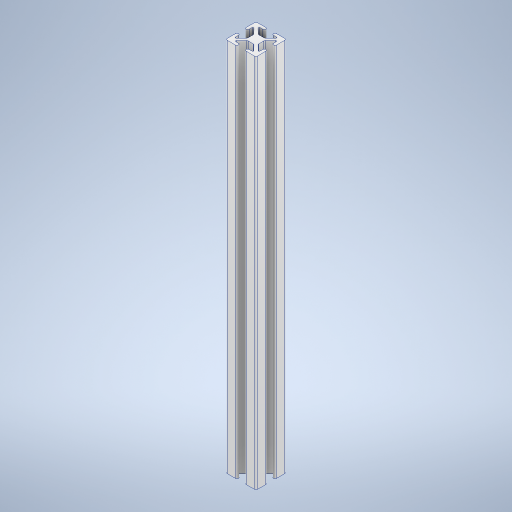
# Autodesk Inventor part: T_slot_1in_12.35in
Saved by Autodesk Inventor 2024 (Build 280153000, 153)
## iProperties
Created: 2024-09-19
Part Number: T_slot_1in_12.35in
Material: Aluminum 6061
Document SubType Name: Modeling
Designer: Owner
Density: 2.7 g/cm^3
Appearance: Aluminum - Flat
Author: Owner
Autodesk Inventor part; units mm, degrees
ref_plane "YZ Plane" through (0, 0, 0) normal (1, 0, 0) x (0, 1, 0)
ref_plane "XZ Plane" through (0, 0, 0) normal (0, 1, 0) x (-1, 0, 0)
ref_plane "XY Plane" through (0, 0, 0) normal (0, 0, 1) x (1, 0, 0)
sketch "Sketch1" plane through (0, 0, 0) normal (0, 1, 0) x (-1, 0, 0)
  line L0 (12.7, 12.7) -> (-12.7, 12.7)
  line L1 (-12.7, 12.7) -> (-12.7, -12.7)
  line L2 (-12.7, -12.7) -> (12.7, -12.7)
  line L3 (12.7, -12.7) -> (12.7, 12.7)
  line L4 (12.7, 12.7) -> (-12.7, -12.7) construction
  line L5 (-12.7, 12.7) -> (12.7, -12.7) construction
  line L6 (10.16, 10.16) -> (-10.16, 10.16)
  line L7 (-10.16, 10.16) -> (-10.16, -10.16)
  line L8 (-10.16, -10.16) -> (10.16, -10.16)
  line L9 (10.16, -10.16) -> (10.16, 10.16)
  line L10 (10.16, 10.16) -> (-10.16, -10.16) construction
  line L11 (-10.16, 10.16) -> (10.16, -10.16) construction
  line L12 (-4.445, 4.445) -> (4.445, 4.445)
  line L13 (4.445, 4.445) -> (4.445, -4.445)
  line L14 (4.445, -4.445) -> (-4.445, -4.445)
  line L15 (-4.445, -4.445) -> (-4.445, 4.445)
  line L16 (-4.445, 4.445) -> (4.445, -4.445) construction
  line L17 (4.445, 4.445) -> (-4.445, -4.445) construction
  line L18 (0, 12.7) -> (-3.175, 12.7)
  line L19 (-3.175, 12.7) -> (3.175, 12.7)
  line L20 (3.175, 12.7) -> (3.175, -12.7)
  line L21 (3.175, -12.7) -> (-3.175, -12.7)
  line L22 (-3.175, -12.7) -> (-3.175, 12.7)
  line L23 (12.7, 0) -> (12.7, 3.175)
  line L24 (12.7, 3.175) -> (-12.7, 3.175)
  line L25 (-12.7, 3.175) -> (-12.7, -3.175)
  line L26 (-12.7, -3.175) -> (12.7, -3.175)
  line L27 (12.7, -3.175) -> (12.7, 3.175)
  line L28 (-13.598, -11.802) -> (11.802, 13.598)
  line L29 (11.802, 13.598) -> (13.598, 11.802)
  line L30 (13.598, 11.802) -> (-11.802, -13.598)
  line L31 (-11.802, -13.598) -> (-13.598, -11.802)
  line L32 (-13.598, -11.802) -> (13.598, 11.802) construction
  line L33 (11.802, 13.598) -> (-11.802, -13.598) construction
  line L34 (-13.598, 11.802) -> (11.802, -13.598)
  line L35 (11.802, -13.598) -> (13.598, -11.802)
  line L36 (13.598, -11.802) -> (-11.802, 13.598)
  line L37 (-11.802, 13.598) -> (-13.598, 11.802)
  line L38 (-13.598, 11.802) -> (13.598, -11.802) construction
  line L39 (11.802, -13.598) -> (-11.802, 13.598) construction
  point P0 (0, 0)
  point P1 (8.3639, 10.16)
  point P2 (2.6489, 4.445)
  point P3 (-2.6489, 4.445)
  point P4 (-8.3639, 10.16)
  point P5 (-10.16, 3.175)
  point P6 (-10.16, 8.3639)
  point P7 (-4.445, 2.6489)
  point P8 (-4.445, -2.6489)
  point P9 (-10.16, -8.3639)
  point P10 (-10.16, -3.175)
  point P11 (-3.175, -10.16)
  point P12 (-8.3639, -10.16)
  point P13 (-2.6489, -4.445)
  point P14 (2.6489, -4.445)
  point P15 (8.3639, -10.16)
  point P16 (3.175, -10.16)
  point P17 (10.16, -3.175)
  point P18 (10.16, -8.3639)
  point P19 (4.445, -2.6489)
  point P20 (4.445, 2.6489)
  point P21 (10.16, 8.3639)
  point P22 (10.16, 3.175)
  point P23 (-3.175, 10.16)
  point P24 (3.175, 10.16)
  dimension "d0" = 25.4
  dimension "d1" = 25.4
  dimension "d2" = 20.32
  dimension "d3" = 20.32
  dimension "d4" = 8.89
  dimension "d5" = 8.89
  dimension "d6" = 3.175
  dimension "d7" = 6.35
  dimension "d8" = 3.175
  dimension "d9" = 6.35
  dimension "d10" = 2.54
  dimension "d11" = 2.54
  constraints: 80 end point, 16 parallel, 12 midpoint, 7 perpendicular, 5 horizontal, 4 point on line
  measures "d0" distance of L2.end L1.end
  measures "d1" distance of L1.end L0.end
  measures "d2" distance of L8.end L7.end
  measures "d3" distance of L7.end L6.end
  measures "d4" distance of L13.end L14.end
  measures "d5" distance of L12.end L13.end
  measures "d6" distance of L18.start L18.end
  measures "d7" distance of L20.end L21.end
  measures "d8" distance of L23.start L23.end
  measures "d9" distance of L25.end L24.end
  measures "d10" distance of L28.end L29.end
  measures "d11" distance of L35.end L34.end
extrude "Extrusion1" add sketch "Sketch1" along normal blind 313.69 contours L0 L28 L6 L20 | L0 L3 L30 L9 L6 L28 | L22 L6 L36 L0 | L6 L9 L30 L24 L13 L12 L20 L28 | L20 L12 L28 | L36 L6 L7 L34 L1 L0 | L3 L24 L9 L30 | L36 L22 L12 L15 L24 L34 L7 L6 | L36 L12 L22 | L20 L24 L28 L12 | L12 L13 L24 L20 | L28 L24 L36 L12 | L22 L24 L15 L12 | L12 L36 L24 L22 | L24 L13 L30 L20 | L20 L30 L36 L28 L24 | L28 L36 L24 | L34 L7 L24 L1 | L30 L13 L24 | L24 L36 L28 L34 L22 | L22 L34 L15 L24 | L30 L13 L36 L20 | L20 L36 L30 | L36 L30 L34 L28 | L3 L36 L9 L26 | L24 L15 L34 | L34 L28 L22 | L22 L28 L15 L34 | L36 L13 L26 L20 | L20 L26 L34 L30 L36 | L34 L30 L26 L22 L28 | L26 L7 L28 L1 | L3 L2 L34 L8 L9 L36 | L9 L8 L34 L20 L14 L13 L26 L36 | L26 L13 L36 | L22 L26 L15 L28 | L26 L13 L14 L20 | L20 L14 L34 L26 | L34 L26 L30 | L28 L7 L8 L30 L2 L1 | L28 L26 L15 L14 L22 L30 L8 L7 | L28 L15 L26 | L26 L30 L14 L22 | L22 L14 L15 L26 | L20 L34 L14 | L34 L14 L30 L26 | L2 L20 L8 L34 | L14 L30 L22 | L30 L8 L22 L2
fillet "Fillet1" radius 1.27 28 edges at (-12.7, 156.845, -12.7) (12.7, 156.845, -12.7) (3.175, 156.845, -12.7) (3.175, 156.845, -10.16) (-3.175, 156.845, -12.7) (-12.7, 156.845, -3.175) (-12.7, 156.845, 3.175) (-10.16, 156.845, 3.175) (-12.7, 156.845, 12.7) (-3.175, 156.845, 10.16) (3.175, 156.845, 12.7) (3.175, 156.845, 10.16) (10.16, 156.845, 3.175) (12.7, 156.845, 3.175) (10.16, 156.845, -3.175) (12.7, 156.845, -3.175) (12.7, 156.845, 12.7) (-3.175, 156.845, -10.16) (-10.16, 156.845, -3.175) (-4.445, 156.845, 2.6489) (-4.445, 156.845, -2.6489) (2.6489, 156.845, -4.445) (-2.6489, 156.845, -4.445) (4.445, 156.845, 2.6489) (4.445, 156.845, -2.6489) (-2.6489, 156.845, 4.445) (2.6489, 156.845, 4.445) (-3.175, 156.845, 12.7)
fillet "Fillet2" radius 0.635 8 edges at (8.3639, 156.845, 10.16) (10.16, 156.845, 8.3639) (-8.3639, 156.845, 10.16) (-10.16, 156.845, 8.3639) (-10.16, 156.845, -8.3639) (-8.3639, 156.845, -10.16) (8.3639, 156.845, -10.16) (10.16, 156.845, -8.3639)
body "Solid1"
